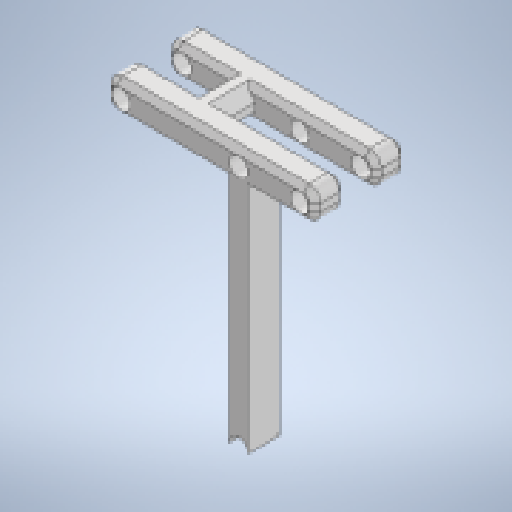
# Autodesk Inventor part: cross-beam
Saved by Autodesk Inventor 2024.1 (Build 281209000, 209)
## iProperties
Created: 2025-07-06
Part Number: cross-beam
Material: Generic
Document SubType Name: Modeling
Designer: iwheard
Density: 1 g/cm^3
Appearance: Default
Author: iwheard
Autodesk Inventor part; units mm, degrees
ref_plane "YZ Plane" through (0, 0, 0) normal (1, 0, 0) x (0, 1, 0)
ref_plane "XZ Plane" through (0, 0, 0) normal (0, 1, 0) x (-1, 0, 0)
ref_plane "XY Plane" through (0, 0, 0) normal (0, 0, 1) x (1, 0, 0)
sketch "Sketch1" plane through (0, 0, 0) normal (0, 0, 1) x (1, 0, 0)
  line L0 (20, 36) -> (-35, 36)
  line L1 (-35, 36) -> (-35, 28)
  line L2 (-35, 28) -> (20, 28)
  line L3 (20, 28) -> (20, 36)
  circle A0 centre (16, 32) radius 2.5
  circle A1 centre (-31, 32) radius 2.5
  arc A2 (-2.5, 32) -> (2.5, 32) centre (0, 32) ccw projected
  line L4 (-2.5, 32) -> (-2.5, -32) projected
  line L5 (2.5, -32) -> (2.5, 32) projected
  arc A3 (2.5, -32) -> (-2.5, -32) centre (0, -32) ccw projected
  arc A4 (0, 34.5) -> (-2.5, 32) centre (0, 32) ccw projected
  arc A5 (2.5, 32) -> (0, 34.5) centre (0, 32) ccw projected
  point P0 (0, 0)
  dimension "d0" = 8
  dimension "d2" = 55
  dimension "d4" = 4
  dimension "d5" = 4
  dimension "d7" = 4
  dimension "d11" = 5
  constraints: 8 end point, 2 centre point, 2 equal radius, 2 parallel, 1 horizontal, 1 horizontal alignment, 1 perpendicular
  measures "d0" distance between parallel lines of L2 L0
  measures "d2" distance between parallel lines of L1 L3
  measures "d4" distance from line of L0 A0.centre
  measures "d5" distance from line of L3 A0.centre
  measures "d7" distance from line of A1.centre L1
  measures "d11" diameter of A1
extrude "Extrusion1" add sketch "Sketch1" along normal blind 8 contours L3 L2 L5 A5 A4 L4 L1 L0 | L5 A3 L4 L2 | L2 L4 A2 L5
fillet "Fillet1" radius 3 4 edges at (-35, 36, 4) (-35, 28, 4) (20, 28, 4) (20, 36, 4)
sketch "Sketch2" plane through (0, 0, 0) normal (0, 0, -1) x (-1, 0, 0)
  arc A0 (-17, 36) -> (-20, 33) centre (-17, 33) ccw projected
  line L0 (-20, 31) -> (-20, 33) projected
  arc A1 (-20, 31) -> (-17, 28) centre (-17, 31) ccw projected
  line L1 (-2.5, 28) -> (-17, 28) projected
  arc A2 (32, 28) -> (35, 31) centre (32, 31) ccw projected
  line L2 (35, 33) -> (35, 31) projected
  arc A3 (35, 33) -> (32, 36) centre (32, 33) ccw projected
  line L3 (-17, 36) -> (32, 36) projected
  line L4 (20, 36) -> (32, 36)
  line L5 (32, 28) -> (20, 28)
  line L6 (20, 28) -> (20, 36)
  line L7 (32, 28) -> (-17, 28) projected
  line L8 (11.5, 36) -> (19.5, 36)
  line L9 (19.5, 36) -> (19.5, 28)
  line L10 (19.5, 28) -> (11.5, 28)
  line L11 (11.5, 28) -> (11.5, 36)
  line L12 (-2.5, -32) -> (-2.5, 28) projected
  arc A4 (2.5, -32) -> (-2.5, -32) centre (0, -32) ccw projected
  line L13 (2.5, 28) -> (2.5, -32) projected
  line L14 (32, 28) -> (2.5, 28) projected
  point P0 (0, 0)
  point P1 (2.5, 28)
  point P2 (-2.5, 28)
  dimension "d12" = 15
  dimension "d21" = 8
  constraints: 14 end point, 3 parallel, 3 point on line, 2 horizontal, 1 perpendicular, 1 point on circle
  measures "d12" distance between parallel lines of L6 L2
  measures "d21" distance between parallel lines of L9 L11
extrude "Extrusion2" add sketch "Sketch2" along normal blind 8 contours L3 L9 L7 L11 | L3 L6 L7 L9
sketch "Sketch3" plane through (0, 0, -8) normal (0, 0, -1) x (-1, 0, 0)
  line L0 (-17, 36) -> (11.5, 36) projected
  arc A0 (-17, 36) -> (-20, 33) centre (-17, 33) ccw projected
  line L1 (-20, 31) -> (-20, 33) projected
  arc A1 (-20, 31) -> (-17, 28) centre (-17, 31) ccw projected
  line L2 (32, 28) -> (19.5, 28) projected
  circle A2 centre (0, 32) radius 2.5 projected
  circle A3 centre (-16, 32) radius 2.5 projected
  line L3 (20, 36) -> (11.5, 36) projected
  line L4 (19.5, 36) -> (19.5, 28) projected
  arc A4 (32, 28) -> (35, 31) centre (32, 31) ccw projected
  line L5 (35, 33) -> (35, 31) projected
  arc A5 (35, 33) -> (32, 36) centre (32, 33) ccw projected
  line L6 (19.5, 36) -> (32, 36) projected
  line L7 (11.5, 28) -> (11.5, 36) projected
  line L8 (11.5, 28) -> (-17, 28) projected
  circle A6 centre (31, 32) radius 2.5 projected
  line L9 (11.5, 28) -> (20, 28) projected
  line L10 (20, 28) -> (20, 36) projected
  line L11 (11.5, 36) -> (11.5, 28) projected
  point P0 (0, 0)
  point P1 (-17, 36)
extrude "Extrusion3" add sketch "Sketch3" along normal blind 8
chamfer "Chamfer1" distance 3 angle 45 4 edges at (-11.5, 36, -4) (-20, 36, -4) (-20, 28, -4) (-11.5, 28, -4)
chamfer "Chamfer2" distance 1.5 angle 45 46 edges at (-13, 36, 0) (2.75, 36, 0) (19.1213, 35.1213, 0) (20, 32, 0) (19.1213, 28.8787, 0) (9.75, 28, 0) (-7, 28, 0) (-13, 28, 0) (-18.5, 36, 0) (-26, 36, 0) (-34.1213, 35.1213, 0) (-35, 32, 0) (-34.1213, 28.8787, 0) (-18.5, 28, 0) (-26, 28, 0) (-18.5, 36, -8) (-26, 36, -8) (-13, 36, -8) (2.75, 36, -8) (-34.1213, 35.1213, -8) (-35, 32, -8) (-34.1213, 28.8787, -8) (2.75, 28, -8) (-13, 28, -8) (-18.5, 28, -8) (-26, 28, -8) (19.1213, 35.1213, -8) (20, 32, -8) (19.1213, 28.8787, -8) (-7.5, 36, -16) (19.1213, 35.1213, -16) (20, 32, -16) (19.1213, 28.8787, -16) (-7.5, 28, -16) (-34.1213, 28.8787, -16) (-35, 32, -16) (-34.1213, 35.1213, -16) (-7.5, 36, 8) (-34.1213, 35.1213, 8) (-35, 32, 8) (-34.1213, 28.8787, 8) (-17.25, 28, 8) (9.75, 28, 8) (19.1213, 28.8787, 8) (20, 32, 8) (19.1213, 35.1213, 8)
